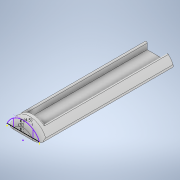
# Autodesk Inventor part: LED arm guard
Saved by Autodesk Inventor 2020 (Build 240168000, 168)
## iProperties
Created: 2021-05-17
Part Number: LED arm guard
Material: Generic
Document SubType Name: Modeling
Designer: Steven
Density: 1 g/cm^3
Appearance: Default
Author: Steven
Autodesk Inventor part; units mm, degrees
ref_plane "YZ Plane" through (0, 0, 0) normal (1, 0, 0) x (0, 1, 0)
ref_plane "XZ Plane" through (0, 0, 0) normal (0, 1, 0) x (-1, 0, 0)
ref_plane "XY Plane" through (0, 0, 0) normal (0, 0, 1) x (1, 0, 0)
sketch "Sketch1" plane through (0, 0, 0) normal (0, 1, 0) x (-1, 0, 0)
  line L0 (0, 0) -> (-15, 0)
  line L1 (-15, 0) -> (-15, -62)
  line L2 (-15, -62) -> (0, -62)
  line L3 (0, -62) -> (0, 0)
  dimension "d0" = 15
  dimension "d1" = 62
  constraints: 8 end point, 2 horizontal, 2 perpendicular
  measures "d0" distance of L0.start L0.end
  measures "d1" distance of L0.end L1.end
extrude "Extrusion1" add sketch "Sketch1" along normal blind 1
sketch "Sketch2" plane through (0, 0, 0) normal (0, 0, 1) x (1, 0, 0)
  line L0 (0, 1) -> (15, 1) construction
  line L1 (7.5, 1) -> (7.5, 6) construction
  arc A0 (15, 1) -> (0, 1) centre (7.5, -2.125) ccw
  line L2 (15, 0) -> (15, 1) projected
  line L3 (0, 1) -> (15, 1)
  line L4 (7.5, 6) -> (12, 6) construction
  line L5 (7.5, 6) -> (3, 6) construction
  line L6 (3, 4.64) -> (3, 1)
  line L7 (12, 4.64) -> (12, 1)
  point P0 (0, 0)
  dimension "d4" = 5
  dimension "d5" = 4.5
  constraints: 12 end point, 5 point on circle, 3 perpendicular, 2 point on line, 1 centre point, 1 horizontal, 1 midpoint, 1 symmetric about line, 1 tangent, 1 vertical
  measures "d4" distance of L1.start L1.end
  measures "d5" distance of L1.end L4.end
extrude "Extrusion2" add sketch "Sketch2" against normal up to surface (62 mm away) contours L3 L7 A0 | L6 L3 A0
extrude "Extrusion3" add sketch "Sketch2" against normal blind 5 contours L7 L3 L6 A0
fillet "Fillet1" radius 0.5 3 edges at (12, 4.64, -33.5) (3, 4.64, -33.5) (7.5, 6, -5)
fillet "Fillet2" radius 3 1 edges at (7.5, 6, 0)
body "Solid1"
